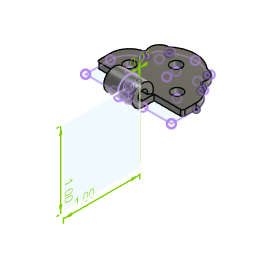
LunchBoxAssembly (Autodesk Fusion 360 archive; units mm, degrees)
design "HingeTop"
Autodesk Fusion 360 part; units mm, degrees
derive "DerivedContext1" from "Hinge Assembly v4"
sketch "Sketch1" plane through (0, 0, 0) normal (0, 0, 1) x (1, 0, 0)
  line L0 (14.2875, 8.2553) -> (14.2875, 0)
  arc A0 (9.2636, 15.3755) -> (9.7459, 14.3423) centre (9.9629, 15.0728) ccw
  arc A1 (9.2636, 15.3755) -> (6.5773, 19.8039) centre (6.35, 16.637) ccw
  arc A2 (6.1406, 19.9814) -> (6.5773, 19.8039) centre (6.6319, 20.5639) ccw
  arc A3 (6.1406, 19.9814) -> (0, 22.225) centre (0, 12.7) ccw
  arc A4 (14.2875, 8.2553) -> (9.7459, 14.3423) centre (7.9375, 8.2553) ccw
  arc A5 (-6.5773, 19.8039) -> (-6.1406, 19.9814) centre (-6.6319, 20.5639) ccw
  arc A6 (-6.5773, 19.8039) -> (-9.2636, 15.3755) centre (-6.35, 16.637) ccw
  arc A7 (-9.7459, 14.3423) -> (-9.2636, 15.3755) centre (-9.9629, 15.0728) ccw
  arc A8 (-9.7459, 14.3423) -> (-14.2875, 8.2553) centre (-7.9375, 8.2553) ccw
  arc A9 (0, 22.225) -> (-6.1406, 19.9814) centre (0, 12.7) ccw
  line L1 (-14.2875, 0) -> (-14.2875, 8.2553)
  line L2 (-14.2875, 0) -> (14.2875, 0)
  point P0 (0, 15.875)
  point P1 (-4.7625, 0)
  point P2 (4.7625, 0)
sketch "Sketch2" plane through (0, 0, 0) normal (1, 0, 0) x (0, 1, 0)
  circle A0 centre (0, 3.4925) radius 3.4925
  circle A1 centre (0, 3.4925) radius 1.5875
  line L0 (0, 3.4925) -> (-3.2819, 2.298)
  line L1 (0, 0) -> (0, 3.4925)
  line L2 (0, 3.4925) -> (3.2819, 2.298)
  constraint symmetric A0.centre L1 A1.centre
  constraint symmetric L0.end L1 L2.end
sketch "sketch 260" plane through (0, 0, 0) normal (0, 0, 1) x (1, 0, 0)
  line L0 (-14.2875, 0) -> (14.2875, 0)
  line L1 (14.2875, -8.2553) -> (14.2875, 0)
  line L2 (-14.2875, 0) -> (-14.2875, -8.2553)
  line L3 (0, 0) -> (0, -22.225) construction
  arc A0 (-6.1406, -19.9814) -> (0, -22.225) centre (0, -12.7) ccw
  arc A1 (-9.2636, -15.3755) -> (-6.5773, -19.8039) centre (-6.35, -16.637) ccw
  arc A2 (-9.2636, -15.3755) -> (-9.7459, -14.3423) centre (-9.9629, -15.0728) ccw
  arc A3 (-6.1406, -19.9814) -> (-6.5773, -19.8039) centre (-6.6319, -20.5639) ccw
  arc A4 (-14.2875, -8.2553) -> (-9.7459, -14.3423) centre (-7.9375, -8.2553) ccw
  arc A5 (9.7459, -14.3423) -> (9.2636, -15.3755) centre (9.9629, -15.0728) ccw
  arc A6 (6.5773, -19.8039) -> (9.2636, -15.3755) centre (6.35, -16.637) ccw
  arc A7 (6.5773, -19.8039) -> (6.1406, -19.9814) centre (6.6319, -20.5639) ccw
  arc A8 (0, -22.225) -> (6.1406, -19.9814) centre (0, -12.7) ccw
  arc A9 (9.7459, -14.3423) -> (14.2875, -8.2553) centre (7.9375, -8.2553) ccw
  arc A10 (-9.7459, 14.3423) -> (-14.2875, 8.2553) centre (-7.9375, 8.2553) ccw
  arc A11 (-9.7459, 14.3423) -> (-9.2636, 15.3755) centre (-9.9629, 15.0728) ccw
  arc A12 (-6.5773, 19.8039) -> (-9.2636, 15.3755) centre (-6.35, 16.637) ccw
  arc A13 (-6.5773, 19.8039) -> (-6.1406, 19.9814) centre (-6.6319, 20.5639) ccw
  arc A14 (0, 22.225) -> (-6.1406, 19.9814) centre (0, 12.7) ccw
  arc A15 (6.1406, 19.9814) -> (6.5773, 19.8039) centre (6.6319, 20.5639) ccw
  arc A16 (9.2636, 15.3755) -> (6.5773, 19.8039) centre (6.35, 16.637) ccw
  arc A17 (9.2636, 15.3755) -> (9.7459, 14.3423) centre (9.9629, 15.0728) ccw
  arc A18 (14.2875, 8.2553) -> (9.7459, 14.3423) centre (7.9375, 8.2553) ccw
  line L4 (14.2875, 8.2553) -> (14.2875, 0)
  line L5 (-14.2875, 0) -> (-14.2875, 8.2553)
  arc A19 (6.1406, 19.9814) -> (0, 22.225) centre (0, 12.7) ccw
  point P0 (-4.7625, 0)
  point P1 (4.7625, 0)
  point P2 (0, -15.875)
  point P3 (0, 15.875)
extrude "Extrude1" add sketch "sketch 260" along normal blind 1.905 contours L0 A10 A11 A12 A13 A14 A15 A16 A17 A18 L4 L5 A19
extrude "Extrude2" add sketch "Sketch2" along normal up to surface (4.7625 mm away) and the other way up to surface (4.7625 mm away) contours A0 A1 L0 L2 | A0 A1 L0 L1
hole "Hole1" at (-7.9375, 8.2553, 0) at (7.9375, 8.2553, 0) at (0, 15.875, 0) direction (0, 0, 1) diameter 3.5814 end up to surface (1.905 mm away)
sketch "Sketch3" plane through (0, 0, 0) normal (1, 0, 0) x (0, 1, 0)
  circle A0 centre (0, 3.4925) radius 3.4925 construction
  line L0 (-21.6535, 3.4925) -> (3.7465, 3.4925)
  line L1 (3.7465, 3.4925) -> (3.7465, -21.9075)
  line L2 (3.7465, -21.9075) -> (-21.6535, -21.9075)
  line L3 (-21.6535, -21.9075) -> (-21.6535, 3.4925)
  line L4 (0, 3.4925) -> (3.4925, 3.4925) construction
  dimension "d9" = 0.254
  dimension "d10" = 25.4
  dimension "d11" = 25.4
  constraint horizontal L0
  constraint vertical L1
  constraint horizontal L2
  constraint vertical L3
  constraint coincident A0.centre L4.start
  constraint coincident A0 L4.end
  constraint horizontal L4
  constraint coincident L0 A0.centre
  measures "d9" distance of L1 L4.end
  measures "d10" distance of L1.end L2.end
  measures "d11" distance of L0.start L2.end
extrude "Extrude3" cut sketch "Sketch3" against normal up to surface (9.525 mm away) from surface at -4.7625
fillet "Fillet1" radius 0.762 1 edges at (-14.2875, 3.7465, 0.9525)
mirror "Mirror1" about plane through (0, 0, 0) normal (1, 0, 0) of "Extrude3", "Fillet1"
equation "d1 = 0.075 \""
equation "d3 = 0.00 \""
equation "d5 = 0.00 \""
equation "d6 = 0.00 °"
equation "d7 = 0.141 \""
equation "d9 = 0.01 \""
equation "d10 = 1\""
equation "d11 = 1\""
equation "d12 = 0.00 \""
equation "d13 = 0.00 \""
equation "d16 = 0.03 \""
equation "d18 = 0.004 \""

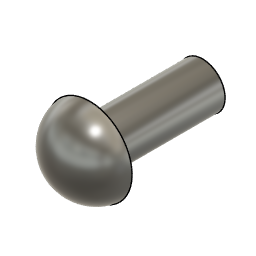
design "Button Head Small Solid Rivet ANSI B18.1.1 - 1/8 x 5/16 Steel Plain"
description: Button Head Small Solid Rivet ANSI B18.1.1 - 1/8 x 5/16
part number: BHSSR ANSI B18.1.1 - 1/8 x 5/16 Steel Plain
Autodesk Fusion 360 part; units mm, degrees
sketch "Sketch1" plane through (0, 0, 0) normal (0, 1, 0) x (1, 0, 0)
  line L0 (-1.5875, 0) -> (-1.5875, 7.9375)
  line L1 (-1.5875, 7.9375) -> (0, 7.9375)
  line L2 (0, 7.9375) -> (0, -2.54)
  line L3 (-1.5875, 0) -> (-2.9845, 0)
  arc A0 (-2.9845, 0) -> (0, -2.54) centre (0, 0.4834) ccw
  dimension "d9" = 3.175
  dimension "d66" = 5.969
  dimension "d106" = 2.54
  dimension "d107" = 7.9375
  constraint perpendicular L0 L1
  constraint collinear origin L2.end L1.end
  constraint perpendicular L0 L3
  constraint coincident origin L3
  constraint vertical L0
  constraint vertical L2
  constraint coincident L2.end A0.end
  constraint coincident L2 A0.centre
  constraint coincident L3.end A0.start
  measures "d106" distance of L3 L2.end
  measures "d107" distance of L1 L3
revolve "Revolve1" add sketch "Sketch1" angle 360 about axis through (0, 0, -7.9375) along (0, 0, 1)
fillet "Fillet4" radius 0.1588 1 edges at (-1.4801, 0.5741, 0)
equation "d9 = adsk_nomdia"
equation "d66 = adsk_headdia"
equation "d100 = adsk_midfillet"
equation "adsk_nomlen = 0.3125 \""
equation "adsk_headh = 0.10 \""
equation "adsk_headdia = 0.235 \""
equation "adsk_nomdia = 0.125 \""
equation "adsk_midfillet = adsk_nomdia * 0.05"
equation "d106 = adsk_headh"
equation "d107 = adsk_nomlen"

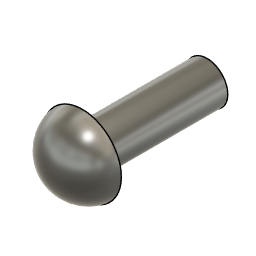
design "Button Head Small Solid Rivet ANSI B18.1.1 - 1/8 x 3/8 Steel Plain"
description: Button Head Small Solid Rivet ANSI B18.1.1 - 1/8 x 3/8
part number: BHSSR ANSI B18.1.1 - 1/8 x 3/8 Steel Plain
Autodesk Fusion 360 part; units mm, degrees
sketch "Sketch1" plane through (0, 0, 0) normal (0, 1, 0) x (1, 0, 0)
  line L0 (-1.5875, 0) -> (-1.5875, 9.525)
  line L1 (-1.5875, 9.525) -> (0, 9.525)
  line L2 (0, 9.525) -> (0, -2.54)
  line L3 (-1.5875, 0) -> (-2.9845, 0)
  arc A0 (-2.9845, 0) -> (0, -2.54) centre (0, 0.4834) ccw
  dimension "d9" = 3.175
  dimension "d66" = 5.969
  dimension "d106" = 2.54
  dimension "d107" = 9.525
  constraint perpendicular L0 L1
  constraint collinear origin L2.end L1.end
  constraint perpendicular L0 L3
  constraint coincident origin L3
  constraint vertical L0
  constraint vertical L2
  constraint coincident L2.end A0.end
  constraint coincident L2 A0.centre
  constraint coincident L3.end A0.start
  measures "d106" distance of L3 L2.end
  measures "d107" distance of L1 L3
revolve "Revolve1" add sketch "Sketch1" angle 360 about axis through (0, 0, -9.525) along (0, 0, 1)
fillet "Fillet4" radius 0.1588 1 edges at (-1.4801, 0.5741, 0)
equation "d9 = adsk_nomdia"
equation "d66 = adsk_headdia"
equation "d100 = adsk_midfillet"
equation "adsk_nomlen = 0.375 \""
equation "adsk_headh = 0.10 \""
equation "adsk_headdia = 0.235 \""
equation "adsk_nomdia = 0.125 \""
equation "adsk_midfillet = adsk_nomdia * 0.05"
equation "d106 = adsk_headh"
equation "d107 = adsk_nomlen"

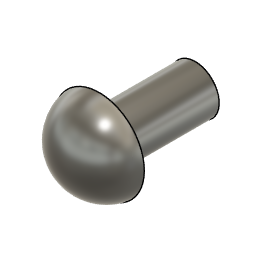
design "Button Head Small Solid Rivet ANSI B18.1.1 - 1/8 x 1/4 Steel Plain"
description: Button Head Small Solid Rivet ANSI B18.1.1 - 1/8 x 1/4
part number: BHSSR ANSI B18.1.1 - 1/8 x 1/4 Steel Plain
Autodesk Fusion 360 part; units mm, degrees
sketch "Sketch1" plane through (0, 0, 0) normal (0, 1, 0) x (1, 0, 0)
  line L0 (-1.5875, 0) -> (-1.5875, 6.35)
  line L1 (-1.5875, 6.35) -> (0, 6.35)
  line L2 (0, 6.35) -> (0, -2.54)
  line L3 (-1.5875, 0) -> (-2.9845, 0)
  arc A0 (-2.9845, 0) -> (0, -2.54) centre (0, 0.4834) ccw
  dimension "d9" = 3.175
  dimension "d66" = 5.969
  dimension "d106" = 2.54
  dimension "d107" = 6.35
  constraint perpendicular L0 L1
  constraint collinear origin L2.end L1.end
  constraint perpendicular L0 L3
  constraint coincident origin L3
  constraint vertical L0
  constraint vertical L2
  constraint coincident L2.end A0.end
  constraint coincident L2 A0.centre
  constraint coincident L3.end A0.start
  measures "d106" distance of L3 L2.end
  measures "d107" distance of L1 L3
revolve "Revolve1" add sketch "Sketch1" angle 360 about axis through (0, 0, -6.35) along (0, 0, 1)
fillet "Fillet4" radius 0.1588 1 edges at (-1.4801, 0.5741, 0)
equation "d9 = adsk_nomdia"
equation "d66 = adsk_headdia"
equation "d100 = adsk_midfillet"
equation "adsk_nomlen = 0.25 \""
equation "adsk_headh = 0.10 \""
equation "adsk_headdia = 0.235 \""
equation "adsk_nomdia = 0.125 \""
equation "adsk_midfillet = adsk_nomdia * 0.05"
equation "d106 = adsk_headh"
equation "d107 = adsk_nomlen"

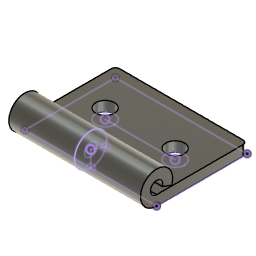
design "Thermos Hinge"
Autodesk Fusion 360 part; units mm, degrees
derive "DerivedContext1" from "Assembly v30"
sketch "Sketch1" plane through (0, 0, 0) normal (0, 0, 1) x (1, 0, 0)
  line L0 (12.7, 7.9375) -> (12.7, -9.525)
  line L1 (12.7, -9.525) -> (-12.7, -9.525)
  line L2 (-12.7, 7.9375) -> (12.7, 7.9375)
  line L3 (-12.7, -9.525) -> (-12.7, 7.9375)
  line L4 (-6.75, 0) -> (6.75, 0)
  circle A0 centre (-6.75, 0) radius 1.7907
  circle A1 centre (6.75, 0) radius 1.7907
sketch "Sketch2" plane through (0, 0, 0) normal (1, 0, 0) x (0, 1, 0)
  circle A0 centre (-9.525, 3.0956) radius 3.0956
  circle A1 centre (-9.525, 3.0956) radius 1.1906
  line L0 (-9.525, 3.0956) -> (-9.525, 0)
  line L1 (-9.525, 3.0956) -> (-6.6161, 2.0369)
extrude "Extrude1" add sketch "Sketch1" along normal blind 1.905
sketch "sketch 596" plane through (0, -93.1403, 61.976) normal (1, 0, 0) x (0, 0, 1)
  line L0 (-61.976, -94.931) -> (-61.976, -91.3496)
  circle A0 centre (-58.8804, -83.6153) radius 3.0956
  circle A1 centre (-58.8804, -83.6153) radius 1.1906
  line L1 (-58.8804, -83.6153) -> (-61.976, -83.6153)
  line L2 (-58.8804, -83.6153) -> (-59.9391, -86.5243)
extrude "Extrude2" add sketch "sketch 596" along normal up to surface (12.7 mm away) and the other way up to surface (12.7 mm away) contours A0 A1 L1 L2 picked at (-60.5276, -81.7964)
fillet "Fillet1" radius 0.7937 2 edges at (-12.7, 7.9375, 0.9525) (12.7, 7.9375, 0.9525)
equation "d1 = 0.075 \""
equation "d3 = 0.00 \""
equation "d5 = 0.00 \""
equation "d6 = 0.00 °"
equation "d8 = 0.03125 \""

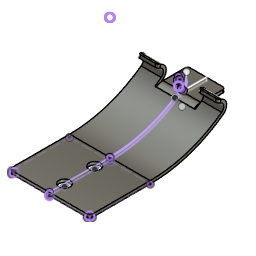
design "Thermos Spring Clip"
Autodesk Fusion 360 part; units mm, degrees
derive "DerivedContext1" from "Assembly v32"
sketch "Sketch1" plane through (0, 0, 0) normal (1, 0, 0) x (0, 1, 0)
  arc A0 (42.1583, 7.5511) -> (41.375, 11.974) centre (40.6809, 9.5703) ccw
  line L0 (41.375, 11.974) -> (40.6429, 12.1854)
  line L1 (40.3892, 11.3069) -> (40.6429, 12.1854)
  line L2 (41.1213, 11.0955) -> (40.3892, 11.3069)
  arc A1 (41.6183, 8.2891) -> (41.1213, 11.0955) centre (40.6809, 9.5703) ccw
  line L3 (0, 0.9144) -> (19.05, 0.9144)
  line L4 (0, 0) -> (0, 0.9144)
  line L5 (0, 0) -> (19.05, 0)
  arc A2 (19.05, 0) -> (42.1583, 7.5511) centre (19.05, 39.134) ccw
  arc A3 (19.05, 0.9144) -> (41.6183, 8.2891) centre (19.05, 39.134) ccw
sketch "sketch 251" plane through (0, -39.3625, 61.976) normal (-1, 0, 0) x (0, 0, -1)
  arc A0 (-25.2151, -1.9704) -> (-24.1375, -1.524) centre (-24.1375, -3.048) cw construction
  line L0 (-24.1375, -1.524) -> (24.1375, -1.524) construction
  arc A1 (24.1375, -1.524) -> (25.2151, -1.9704) centre (24.1375, -3.048) cw construction
  line L1 (25.2151, -1.9704) -> (61.5296, -38.2849) construction
  arc A2 (61.5296, -38.2849) -> (61.976, -39.3625) centre (60.452, -39.3625) cw construction
  line L2 (61.976, -101.6) -> (63.5, -101.6) construction
  arc A3 (63.5, -39.3625) -> (62.6073, -37.2073) centre (60.452, -39.3625) ccw construction
  line L3 (62.6073, -37.2073) -> (26.2927, -0.8927) construction
  arc A4 (26.2927, -0.8927) -> (24.1375, 0) centre (24.1375, -3.048) ccw construction
  line L4 (24.1375, 0) -> (-24.1375, 0) construction
  arc A5 (-24.1375, 0) -> (-26.2927, -0.8927) centre (-24.1375, -3.048) ccw construction
  line L5 (-26.2927, -0.8927) -> (-62.6073, -37.2073) construction
  arc A6 (-62.6073, -37.2073) -> (-63.5, -39.3625) centre (-60.452, -39.3625) ccw construction
  line L6 (-63.5, -39.3625) -> (-63.5, -101.6) construction
  line L7 (-63.5, -101.6) -> (-61.976, -101.6) construction
  line L8 (-61.976, -101.6) -> (-61.976, -39.3625) construction
  arc A7 (-61.976, -39.3625) -> (-61.5296, -38.2849) centre (-60.452, -39.3625) cw construction
  line L9 (-61.5296, -38.2849) -> (-25.2151, -1.9704) construction
  arc A8 (-59.2876, -84.7342) -> (-60.071, -83.6153) centre (-58.8804, -83.6153) ccw construction
  circle A9 centre (0, -45.974) radius 44.45 construction
  circle A10 centre (-58.8804, -83.6153) radius 1.1906
  line L10 (-58.8804, -83.6153) -> (61.976, -83.6153) construction
  line L11 (-58.8804, -83.6153) -> (-40.1584, -87.1355)
  arc A11 (-40.1584, -87.1355) -> (33.9149, -85.0222) centre (-7.975, 84.0302) ccw
  circle A12 centre (52.4057, -80.4403) radius 1.1906 construction
  line L12 (33.9149, -85.0222) -> (52.4057, -80.4403)
  line L13 (105.9485, -108.8525) -> (89.8425, -89.319) construction
  line L14 (89.8425, -89.319) -> (89.8425, -78.7171) construction
  line L15 (89.8425, -78.7171) -> (106.7144, -78.7171) construction
  circle A13 centre (0, -45.974) radius 45.6406 construction
  line L16 (0, -45.974) -> (0, 0) construction
  circle A14 centre (-58.8804, -83.6153) radius 111.3314 construction
  line L17 (-40.1584, -87.1355) -> (33.9149, -85.0222) construction
  line L18 (59.557, 1769.7758) -> (58.3378, 1769.7758)
  line L19 (52.4057, -80.4403) -> (52.4057, -73.7437) construction
  arc A15 (53.6869, -80.9809) -> (61.0616, -58.4125) centre (22.842, -58.4125) ccw
  arc A16 (54.4249, -81.5208) -> (61.976, -58.4125) centre (22.842, -58.4125) ccw
  line L20 (61.976, -39.3625) -> (61.0616, -39.3625)
  line L21 (61.0616, -39.3625) -> (61.0616, -58.4125)
  line L22 (61.976, -39.3625) -> (61.976, -58.4125)
  arc A17 (52.4057, -78.456) -> (52.3315, -78.4577) centre (52.4057, -80.0435) ccw
  arc A18 (50.8805, -80.4839) -> (53.6869, -80.9809) centre (52.4057, -80.0435) ccw
  arc A19 (50.002, -80.7375) -> (54.4249, -81.5208) centre (52.4057, -80.0435) ccw
  line L23 (52.4057, -80.4403) -> (-58.8804, -83.6153) construction
  line L24 (52.4057, -80.0435) -> (50.002, -80.7375)
  line L25 (50.8805, -80.4839) -> (50.6691, -79.7518)
  line L26 (50.002, -80.7375) -> (49.7906, -80.0054)
  line L27 (50.6691, -79.7518) -> (49.7906, -80.0054)
  circle A20 centre (61.976, -58.4125) radius 24.1497 construction
  line L28 (63.5, -55.4407) -> (61.976, -55.4407)
  line L29 (61.976, -55.4407) -> (61.976, -101.6)
  line L30 (63.5, -101.6) -> (63.5, -55.4407)
  line L31 (63.5, -45.9157) -> (61.976, -45.9157)
  line L32 (61.976, -45.9157) -> (61.976, -51.8593)
  line L33 (61.976, -51.8593) -> (63.5, -51.8593)
  line L34 (63.5, -51.8593) -> (63.5, -45.9157)
  line L35 (61.976, -39.3625) -> (61.976, -42.3343)
  line L36 (61.976, -42.3343) -> (63.5, -42.3343)
  line L37 (63.5, -42.3343) -> (63.5, -39.3625)
  point P0 (52.451, -83.6153)
  point P1 (-3.0081, -90.0641)
extrude "Extrude1" add sketch "sketch 251" along normal mid plane 25.4 contours L12 A18 A19 L24 | L12 A15 A16 L20 L21 L22 A18 A19 L29 L32 L35 | L24 L25 L26 L27
sketch "Sketch2" plane through (0, 0, 0) normal (1, 0, 0) x (0, 1, 0)
  arc A0 (19.05, 0) -> (42.1583, 7.5511) centre (19.05, 39.134) ccw
  arc A1 (19.05, 0.9144) -> (41.6183, 8.2891) centre (19.05, 39.134) ccw
  arc A2 (42.1583, 7.5511) -> (41.375, 11.974) centre (40.6809, 9.5703) ccw
  arc A3 (42.1583, 7.5511) -> (41.375, 11.974) centre (40.6809, 9.5703) ccw
  arc A4 (41.6183, 8.2891) -> (41.1213, 11.0955) centre (40.6809, 9.5703) ccw
  line L0 (41.7995, 7.5511) -> (49.5328, 7.5511)
  line L1 (49.5328, 7.5511) -> (49.5328, 6.6367)
  line L2 (49.5328, 6.6367) -> (41.7995, 6.6367)
  arc A5 (41.7995, 6.6367) -> (40.0923, 6.1387) centre (41.7995, 3.4617) ccw
  arc A6 (19.05, 0) -> (42.1583, 7.5511) centre (19.05, 39.134) ccw
  arc A7 (19.05, 0.9144) -> (41.6183, 8.2891) centre (19.05, 39.134) ccw
  arc A8 (19.05, 0.9144) -> (41.6183, 8.2891) centre (19.05, 39.134) ccw
  arc A9 (41.7995, 7.5511) -> (39.6007, 6.9097) centre (41.7995, 3.4617) ccw
  line L3 (40.3892, 11.3069) -> (40.6429, 12.1854)
  line L4 (43.1828, 6.6367) -> (43.1828, 12.1876) construction
  arc A10 (42.1583, 7.5511) -> (41.375, 11.974) centre (40.6809, 9.5703) ccw
  line L5 (40.0923, 6.1387) -> (39.6007, 6.9097)
  line L6 (41.1213, 11.0955) -> (40.3892, 11.3069)
  line L7 (40.3892, 11.3069) -> (40.6429, 12.1854)
  line L8 (41.375, 11.974) -> (40.6429, 12.1854)
  point P0 (42.1583, 7.5511)
  dimension "d4" = 6.35
  dimension "d5" = 3.175
  constraint horizontal L0
  constraint perpendicular L0 L1
  constraint perpendicular L1 L2
  constraint tangent L2 A5
  constraint coincident A0 A5.end
  constraint tangent A5 A6
  constraint concentric A5 A9
  constraint tangent A8 A9
  constraint equal L1 L3
  constraint coincident A1 A9.end
  constraint coincident L2 L4.start
  constraint perpendicular L2 L4
  constraint tangent L4 A10
  constraint coincident L0 P0
  measures "d4" distance of L1 L4
  measures "d5" radius of A5
extrude "Extrude2" cut sketch "Sketch2" along normal mid plane 12.7 contours A0 L0 A6 A9 L5 | A1 A2 A3 A4 L0 A7 A8 A9 L3 A10 L6 L7 L8
extrude "Extrude3" add sketch "Sketch2" along normal mid plane 11.9062 contours A0 L0 A6 A9 L5 | A0 L0 L1 L2 A5 A6
fillet "Fillet1" radius 0.7937 8 edges at (5.9531, 49.5328, 7.0939) (-5.9531, 49.5328, 7.0939) (-12.7, 40.5161, 11.7461) (-6.35, 40.5161, 11.7461) (6.35, 40.5161, 11.7461) (12.7, 40.5161, 11.7461) (12.7, 0, 0.4572) (-12.7, 0, 0.4572)
sketch "Sketch3" plane through (0, 0, 0) normal (0, 0, 1) x (1, 0, 0)
  arc A0 (-12.7, 0.7938) -> (-11.9062, 0) centre (-11.9062, 0.7938) ccw construction
  line L0 (-12.7, 0.7938) -> (-12.7, 19.05) construction
  line L1 (-12.7, 19.05) -> (12.7, 19.05) construction
  line L2 (12.7, 19.05) -> (12.7, 0.7938) construction
  arc A1 (11.9062, 0) -> (12.7, 0.7938) centre (11.9062, 0.7938) ccw construction
  line L3 (11.9062, 0) -> (-11.9062, 0) construction
  line L4 (0, 0) -> (0, 19.05) construction
  point P0 (0, 4.7625)
  point P1 (0, 14.2875)
  dimension "d12" = 4.7625
  dimension "d13" = 4.7625
  constraint coincident L4 P0
  constraint coincident L4 P1
  measures "d12" distance of L1 P1
  measures "d13" distance of L3 P0
hole "Hole1" at (0, 14.2875, 0) at (0, 4.7625, 0) direction (0, 0, 1) diameter 3.5814 depth 1.524 tip angle 118
equation "d1 = 1\""
equation "d4 = 0.25 \""
equation "d5 = 0.125 \""
equation "d6 = 0.5 \""
equation "d8 = 0.5 \" - 0.03125 \""
equation "d11 = 0.03125 \""
equation "d12 = d13"
equation "d13 = 0.1875 \""
equation "d14 = 0.06 \""
equation "d15 = 0.141 \""

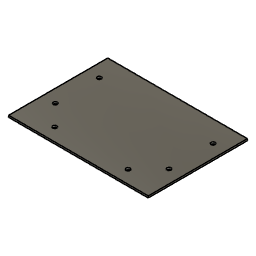
design "Bottom Side Panel" references "parameters"
Autodesk Fusion 360 part; units mm, degrees
derive "DerivedContext3" from "Base Assembly v6"
sketch "Sketch1" plane through (0, 0, 0) normal (0, 0, 1) x (1, 0, 0)
  line L0 (-60.452, 44.45) -> (60.452, 44.45)
  line L1 (60.452, 44.45) -> (60.452, -41.402)
  line L2 (60.452, -41.402) -> (-60.452, -41.402)
  line L3 (-60.452, -41.402) -> (-60.452, 44.45)
  point P0 (60.452, -40.3244)
  point P1 (59.3744, -41.402)
  point P2 (-60.452, 44.45)
  point P3 (-49.2125, 25.9388)
  point P4 (-49.2125, -12.1612)
  point P5 (-31.75, -30.1625)
  point P6 (31.75, -30.1625)
  point P7 (49.2125, -12.1612)
  point P8 (49.2125, 25.9388)
  constraint horizontal L0
  constraint vertical L1
  constraint horizontal L2
  constraint vertical L3
  constraint coincident P2 L0.start
  constraint coincident L2 P1
  constraint coincident L1 P0
derive "Derived from parameters v2" from "parameters v2"
extrude "Extrude1" add sketch "Sketch1" along normal blind 1.524
hole "Hole1" at (-49.2125, 25.9388, 0) at (-49.2125, -12.1612, 0) at (-31.75, -30.1625, 0) at (31.75, -30.1625, 0) at (49.2125, -12.1612, 0) at (49.2125, 25.9388, 0) direction (0, 0, 1) diameter 3.5717 end up to surface (1.524 mm away)
equation "d1 = 0.10 \""
equation "thickness_Ref = 0.06 \""
equation "radius_Ref = 0.066 \""
equation "width_Ref = 5\""
equation "length_Ref = 12\""
equation "bottomHeight_Ref = 3.5 \""
equation "topHeight_Ref = 4\""
equation "topWidth_Ref = 2\""
equation "topAngle_Ref = 45 °"
equation "d10 = thickness_Ref"
equation "d12 = 0.125 \" + 0.01562 \""

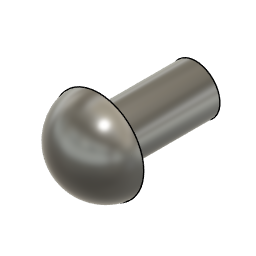
design "Button Head Small Solid Rivet ANSI B18.1.1 - 5/32 x 5/16 Steel Plain"
description: Button Head Small Solid Rivet ANSI B18.1.1 - 5/32 x 5/16
part number: BHSSR ANSI B18.1.1 - 5/32 x 5/16 Steel Plain
Autodesk Fusion 360 part; units mm, degrees
sketch "Sketch1" plane through (0, 0, 0) normal (0, 1, 0) x (1, 0, 0)
  line L0 (-1.9844, 0) -> (-1.9844, 7.9375)
  line L1 (-1.9844, 7.9375) -> (0, 7.9375)
  line L2 (0, 7.9375) -> (0, -3.1496)
  line L3 (-1.9844, 0) -> (-3.683, 0)
  arc A0 (-3.683, 0) -> (0, -3.1496) centre (0, 0.5786) ccw
  dimension "d9" = 3.9688
  dimension "d66" = 7.366
  dimension "d106" = 3.1496
  dimension "d107" = 7.9375
  constraint perpendicular L0 L1
  constraint collinear origin L2.end L1.end
  constraint perpendicular L0 L3
  constraint coincident origin L3
  constraint vertical L0
  constraint vertical L2
  constraint coincident L2.end A0.end
  constraint coincident L2 A0.centre
  constraint coincident L3.end A0.start
  measures "d106" distance of L3 L2.end
  measures "d107" distance of L1 L3
revolve "Revolve1" add sketch "Sketch1" angle 360 about axis through (0, 0, -7.9375) along (0, 0, 1)
fillet "Fillet4" radius 0.1984 1 edges at (-1.8501, 0.7176, 0)
equation "d9 = adsk_nomdia"
equation "d66 = adsk_headdia"
equation "d100 = adsk_midfillet"
equation "adsk_nomlen = 0.3125 \""
equation "adsk_headh = 0.124 \""
equation "adsk_headdia = 0.29 \""
equation "adsk_nomdia = 0.15625 \""
equation "adsk_midfillet = adsk_nomdia * 0.05"
equation "d106 = adsk_headh"
equation "d107 = adsk_nomlen"
